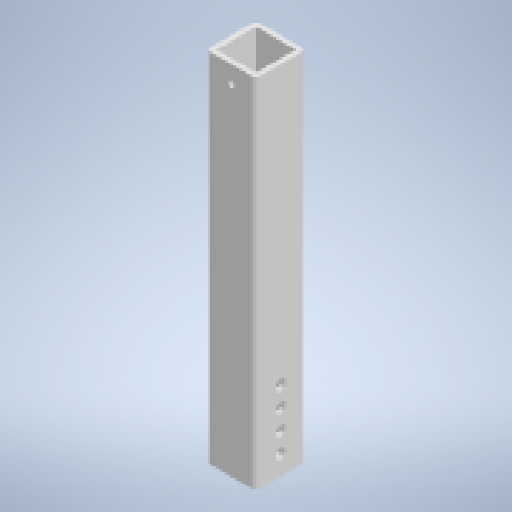
# Autodesk Inventor part: suspension2chassisarm
Saved by Autodesk Inventor 2025.2 (Build 292293000, 293)
## iProperties
Created: 2026-03-19
Part Number: suspension2chassisarm
Material: Generic
Document SubType Name: Modeling
Designer: hp
Density: 1 g/cm^3
Appearance: Default
Author: hp
Autodesk Inventor part; units mm, degrees
ref_plane "YZ Plane" through (0, 0, 0) normal (1, 0, 0) x (0, 1, 0)
ref_plane "XZ Plane" through (0, 0, 0) normal (0, 1, 0) x (-1, 0, 0)
ref_plane "XY Plane" through (0, 0, 0) normal (0, 0, 1) x (1, 0, 0)
sketch "Sketch1" plane through (0, 0, 0) normal (0, 1, 0) x (-1, 0, 0)
  line L0 (8, 10) -> (-8, 10)
  line L1 (-10, 8) -> (-10, -8)
  line L2 (-8, -10) -> (8, -10)
  line L3 (10, -8) -> (10, 8)
  line L4 (10, 10) -> (-10, -10) construction
  line L5 (-10, 10) -> (10, -10) construction
  line L6 (8, 8) -> (-8, 8)
  line L7 (-8, 8) -> (-8, -8)
  line L8 (-8, -8) -> (8, -8)
  line L9 (8, -8) -> (8, 8)
  arc A0 (10, 8) -> (8, 10) centre (8, 8) ccw
  arc A1 (8, -10) -> (10, -8) centre (8, -8) ccw
  arc A2 (-10, -8) -> (-8, -10) centre (-8, -8) ccw
  arc A3 (-8, 10) -> (-10, 8) centre (-8, 8) ccw
  point P0 (0, 0)
  dimension "d0" = 20
  dimension "d1" = 20
  dimension "d2" = 2
  dimension "d3" = 2
  dimension "d4" = 2
  constraints: 20 end point, 8 point on circle, 8 point on line, 8 tangent, 4 centre point, 4 parallel, 2 equal radius, 2 midpoint, 2 perpendicular, 1 horizontal, 3 other
  measures "d0" distance of L5.end L4.end
  measures "d1" distance of L4.end L5.start
  measures "d2" distance between parallel lines of L3 L9
  measures "d3" radius of A0
  measures "d4" radius of A3
extrude "Extrusion1" add sketch "Sketch1" along normal blind 144
sketch "Sketch2" plane through (10, 0, 8) normal (1, 0, 0) x (0, 0, -1)
  line L0 (0, 0) -> (16, 0) projected
  line L1 (16, 0) -> (16, 144) projected
  point P0 (8, 0)
  point P1 (8, 8)
  point P2 (8, 0)
  point P3 (8, 16)
  point P4 (8, 24)
  point P5 (8, 32)
  dimension "d7" = 8
  dimension "d10" = 8
  constraints: 1 midpoint, 1 vertical, 3 other
  measures "d7" distance of point (8, 0) point (8, 8)
  measures "d10" distance of point (8, 8) point (8, 16)
hole "Hole1" at (10, 8, 0) at (10, 16, 0) at (10, 24, 0) at (10, 32, 0) direction (-1, 0, 0) diameter 4.05 end through all
sketch "Sketch3" plane through (-8, 0, 10) normal (0, 0, 1) x (1, 0, 0)
  line L0 (0, 144) -> (16, 144) projected
  line L1 (0, 0) -> (0, 144) projected
  point P0 (8, 0)
  point P1 (8, 135)
  point P2 (8, 144)
  dimension "d22" = 9
  dimension "d23" = 8
  constraints: 1 midpoint
  measures "d22" distance of point (8, 144) point (8, 135)
  measures "d23" distance from line of point (8, 135) L1
hole "Hole2" at (0, 135, 10) direction (0, 0, -1) diameter 2.45 depth 2
body "Solid1"
